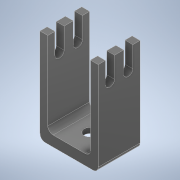
# Autodesk Inventor part: magnetsupport
Saved by Autodesk Inventor 2022 (Build 260153000, 153)
## iProperties
Created: 2022-08-13
Part Number: magnetsupport
Material: Genérico
Document SubType Name: Modeling
Designer: JK
Density: 1 g/cm^3
Appearance: Suave - Negro
Author: JK
Autodesk Inventor part; units mm, degrees
ref_plane "YZ Plane" through (0, 0, 0) normal (1, 0, 0) x (0, 1, 0)
ref_plane "XZ Plane" through (0, 0, 0) normal (0, 1, 0) x (-1, 0, 0)
ref_plane "XY Plane" through (0, 0, 0) normal (0, 0, 1) x (1, 0, 0)
sketch "Boceto1" plane through (0, 0, 0) normal (0, 1, 0) x (-1, 0, 0)
  circle A0 centre (0, 0) radius 2.25
  line L0 (-8.15, 8) -> (8.15, 8)
  line L1 (8.15, 8) -> (8.15, -8)
  line L2 (8.15, -8) -> (-8.15, -8)
  line L3 (-8.15, -8) -> (-8.15, 8)
  line L4 (-8.15, 8) -> (8.15, -8) construction
  line L5 (8.15, 8) -> (-8.15, -8) construction
  dimension "d0" = 4.5
  dimension "d1" = 16.3
  dimension "d2" = 16
  constraints: 12 end point, 2 midpoint, 2 parallel, 1 centre point, 1 coincident, 1 horizontal, 1 perpendicular
  measures "d0" diameter of A0
  measures "d1" distance of L1.end L2.end
  measures "d2" distance of L0.end L1.end
extrude "Extrusión1" add sketch "Boceto1" along normal blind 4
sketch "Boceto3" plane through (0, 0, 0) normal (0, -1, 0) x (1, 0, 0)
  line L0 (11.15, 8) -> (-11.15, 8)
  line L1 (-11.15, 8) -> (-11.15, -8)
  line L2 (-11.15, -8) -> (11.15, -8)
  line L3 (11.15, -8) -> (11.15, 8)
  circle A0 centre (0, 0) radius 2.25 projected
  line L4 (11.15, 8) -> (-11.15, -8) construction
  line L5 (-11.15, 8) -> (11.15, -8) construction
  line L6 (8.15, -8) -> (-8.15, -8) projected
  line L7 (8.15, 8) -> (8.15, -8) projected
  line L8 (8.15, -8) -> (-8.15, -8) projected
  line L9 (8.15, 8) -> (8.15, -8) projected
  line L10 (-8.15, 8) -> (8.15, 8) projected
  line L11 (-8.15, -8) -> (-8.15, 8) projected
  circle A1 centre (0, 0) radius 2.25 projected
  point P0 (-8.15, 8)
  dimension "d8" = 3
  constraints: 12 end point, 2 midpoint, 2 parallel, 1 collinear, 1 horizontal, 1 perpendicular
  measures "d8" distance between parallel lines of L7 L3
extrude "Extrusión3" add sketch "Boceto3" against normal blind 36 contours L3 L2 L7 L0 | L11 L2 L1 L0
sketch "Boceto4" plane through (11.15, 0, 8) normal (1, 0, 0) x (0, 0, -1)
  circle A0 centre (4.5, 28) radius 1.75
  circle A1 centre (11.5, 28) radius 1.75
  line L0 (0, 36) -> (16, 36) projected
  line L1 (0, 0) -> (0, 36) projected
  line L2 (2.75, 36) -> (6.25, 36)
  line L3 (6.25, 36) -> (6.25, 28)
  line L4 (6.25, 28) -> (2.75, 28)
  line L5 (2.75, 28) -> (2.75, 36)
  line L6 (9.75, 36) -> (13.25, 36)
  line L7 (13.25, 36) -> (13.25, 28)
  line L8 (13.25, 28) -> (9.75, 28)
  line L9 (9.75, 28) -> (9.75, 36)
  point P0 (8, 0)
  point P1 (9.75, 28)
  point P2 (13.25, 36)
  dimension "d11" = 8
  dimension "d12" = 3.5
  dimension "d14" = 7
  dimension "d18" = 4.5
  constraints: 16 end point, 4 parallel, 2 collinear, 2 horizontal, 2 perpendicular, 2 tangent, 2 vertical, 1 centre point, 1 horizontal alignment, 1 point on line, 4 other
  measures "d11" distance from line of L0 A1.centre
  measures "d12" diameter of A1
  measures "d14" distance of A1.centre point (4.5, 28)
  measures "d18" distance from line of L1 point (4.5, 28)
extrude "Extrusión4" cut sketch "Boceto4" against normal through all
fillet "Empalme1" radius 2 2 edges at (-11.15, 0, 0) (11.15, 0, 0)
sketch "Boceto6" plane through (0, 0, 0) normal (0, -1, 0) x (1, 0, 0)
  circle A0 centre (0, 0) radius 5
  dimension "d24" = 10
  constraints: 1 centre point, 1 coincident
  measures "d24" diameter of A0
extrude "Extrusión6" cut sketch "Boceto6" against normal blind 2
fillet "Empalme2" radius 2 2 edges at (-8.15, 4, 0) (8.15, 4, 0)
sketch "Boceto5" plane through (-11.15, 28, 5.25) normal (-1, 0, 0) x (0, 0, 1)
  arc A0 (-10.5, 0) -> (-7, 0) centre (-8.75, 0) ccw projected
  circle A1 centre (-8.75, 0) radius 2.85
  arc A2 (-3.5, 0) -> (0, 0) centre (-1.75, 0) ccw projected
  circle A3 centre (-1.75, 0) radius 2.85
  line L0 (-11.6, 0) -> (-5.9, 0)
  line L1 (-5.9, 0) -> (-5.9, 8.628)
  line L2 (-5.9, 8.628) -> (-11.6, 8.628)
  line L3 (-11.6, 8.628) -> (-11.6, 0)
  line L4 (-4.6, 0) -> (1.1, 0)
  line L5 (1.1, 0) -> (1.1, 8.628)
  line L6 (1.1, 8.628) -> (-4.6, 8.628)
  line L7 (-4.6, 8.628) -> (-4.6, 0)
  line L8 (-8.75, 3.2909) -> (-5.9, 1.6454)
  line L9 (-5.9, 1.6454) -> (-5.9, -1.6454)
  line L10 (-5.9, -1.6454) -> (-8.75, -3.2909)
  line L11 (-8.75, -3.2909) -> (-11.6, -1.6454)
  line L12 (-11.6, -1.6454) -> (-11.6, 1.6454)
  line L13 (-11.6, 1.6454) -> (-8.75, 3.2909)
  line L14 (-1.75, 3.2909) -> (1.1, 1.6454)
  line L15 (1.1, 1.6454) -> (1.1, -1.6454)
  line L16 (1.1, -1.6454) -> (-1.75, -3.2909)
  line L17 (-1.75, -3.2909) -> (-4.6, -1.6454)
  line L18 (-4.6, -1.6454) -> (-4.6, 1.6454)
  line L19 (-4.6, 1.6454) -> (-1.75, 3.2909)
  point P0 (-5.25, -28)
  point P1 (0, 0)
  point P2 (-3.5, 0)
  point P3 (1.1, 0)
  point P4 (-10.5, 0)
  point P5 (-7.325, -2.4682)
  point P6 (-10.175, -2.4682)
  point P7 (-11.6, 0)
  point P8 (-3.175, -2.4682)
  point P9 (-0.325, -2.4682)
  point P10 (1.1, 0)
  dimension "d20" = 5.7
  dimension "d21" = 5.7
  constraints: 40 end point, 6 vertical, 4 coincident, 4 parallel, 2 horizontal, 2 perpendicular, 2 vertical alignment, 1 point on line, 32 other
